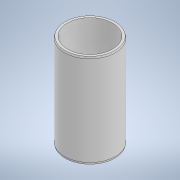
# Autodesk Inventor part: 75. Втулка блока заднего хода
Saved by Autodesk Inventor 2021 (Build 250183000, 183)
## iProperties
Created: 2021-03-15
Part Number: 75. Втулка блока заднего хода
Material: Типовые
Document SubType Name: Modeling
Designer: Данил
Density: 1 g/cm^3
Appearance: По умолчанию
Author: Данил
Autodesk Inventor part; units mm, degrees
ref_plane "YZ Plane" through (0, 0, 0) normal (1, 0, 0) x (0, 1, 0)
ref_plane "XZ Plane" through (0, 0, 0) normal (0, 1, 0) x (-1, 0, 0)
ref_plane "XY Plane" through (0, 0, 0) normal (0, 0, 1) x (1, 0, 0)
sketch "Эскиз1" plane through (0, 0, 0) normal (0, 0, 1) x (1, 0, 0)
  line L0 (0, 26) -> (0, -26)
  line L1 (12.573, 26) -> (13.8571, 26)
  line L2 (14.125, 25) -> (14.125, -25)
  line L3 (13.8571, -26) -> (12.573, -26)
  line L4 (12.573, -26) -> (12.573, 26)
  line L5 (14.125, 25) -> (13.8571, 26)
  line L6 (14.125, -25) -> (13.8571, -26)
  point P0 (0, 0)
  point P1 (0, 0)
  point P2 (14.125, -26)
  point P3 (14.125, 26)
  dimension "d0" = 52
  dimension "d1" = 28.25
  dimension "d2" = 25.146
  dimension "d3" = 1
  dimension "d4" = 15
  dimension "d5" = 1
  dimension "d6" = 15
  constraints: 14 end point, 4 point on line, 2 horizontal alignment, 2 parallel, 1 coincident, 1 horizontal, 1 midpoint, 1 perpendicular, 1 vertical
  measures "d0" distance of L0.start L0.end
  measures "d1" diameter of L2 L0
  measures "d2" diameter of L4 L0
  measures "d3" distance of L2.start point (14.125, 26)
  measures "d4" angle of L2 L5
  measures "d5" distance of L2.end point (14.125, -26)
  measures "d6" angle of L2 L6
revolve "Вращение1" add sketch "Эскиз1" angle 360 about axis through (0, 26, 0) along (0, -1, 0)
equation "\"d5\" = d3"
equation "\"d6\" = d4"
